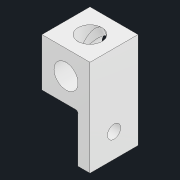
# Autodesk Inventor part: scara-base9
Saved by Autodesk Inventor 2022 (Build 260153000, 153)
## iProperties
Created: 2021-10-21
Part Number: scara-base9
Material: ABS プラスチック
Document SubType Name: Modeling
Designer: Yuta Kage
Density: 1.06 g/cm^3
Appearance: 滑らか - 白
Author: Yuta Kage
Autodesk Inventor part; units mm, degrees
ref_plane "YZ Plane" through (0, 0, 0) normal (1, 0, 0) x (0, 1, 0)
ref_plane "XZ Plane" through (0, 0, 0) normal (0, 1, 0) x (-1, 0, 0)
ref_plane "XY Plane" through (0, 0, 0) normal (0, 0, 1) x (1, 0, 0)
sketch "スケッチ4" plane through (0, 0, 0) normal (0, 0, 1) x (1, 0, 0)
  line L0 (0, 0) -> (0, 40)
  line L1 (0, 40) -> (-20, 40)
  line L2 (-20, 40) -> (-20, 20)
  line L3 (-20, 20) -> (-5, 20)
  line L4 (-5, 20) -> (-5, 0)
  line L5 (-5, 0) -> (0, 0)
  dimension "d32" = 20
  dimension "d33" = 20
  dimension "d34" = 5
  dimension "d58" = 20
  constraints: 12 end point, 5 perpendicular, 1 vertical
  measures "d32" distance of L3.end L4.end
  measures "d33" distance of L1.end L2.end
  measures "d34" distance between parallel lines of L0 L4
  measures "d58" distance of L0.end L1.end
extrude "押し出し2" add sketch "スケッチ4" along normal mid plane 20
sketch "スケッチ5" plane through (0, 0, 10) normal (1, 0, 0) x (0, 0, -1)
  line L0 (20, 0) -> (0, 0) projected
  point P0 (10, 0)
  point P1 (10, 10)
  point P2 (10, 0)
  dimension "d38" = 10
  constraints: 1 midpoint, 1 vertical alignment
  measures "d38" distance of point (10, 0) point (10, 10)
hole "穴3" at (0, 10, 0) direction (-1, 0, 0) diameter 5.5 end through all clearance for "Socket Head Cap Screw" size "M5" standard "Ansi Metric M Profile"
fillet "フィレット3" radius 1 1 edges at (-5, 20, 0)
sketch "スケッチ6" plane through (-20, 40, 10) normal (0, 1, 0) x (1, 0, 0)
  circle A0 centre (10, 10) radius 5
  line L0 (0, 20) -> (0, 0) projected
  line L1 (20, 0) -> (20, 20) projected
  point P0 (20, 10)
  point P1 (20, 10)
  dimension "d47" = 10
  dimension "d48" = 10
  constraints: 1 centre point, 1 horizontal alignment, 1 midpoint
  measures "d47" diameter of A0
  measures "d48" distance from line of L0 A0.centre
extrude "押し出し3" cut sketch "スケッチ6" against normal blind 10
sketch "スケッチ8" plane through (0, 0, 10) normal (0, 0, 1) x (1, 0, 0)
  circle A0 centre (-10, 30) radius 5
  line L0 (0, 40) -> (-20, 40) projected
  line L1 (-20, 40) -> (-20, 20) projected
  point P0 (0, 0)
  dimension "d59" = 10
  dimension "d60" = 10
  dimension "d61" = 10
  constraints: 1 centre point
  measures "d59" diameter of A0
  measures "d60" distance from line of A0.centre L0
  measures "d61" distance from line of L1 A0.centre
extrude "押し出し5" cut sketch "スケッチ8" against normal blind 20
fillet "フィレット6" radius 5 4 edges at (-6.4645, 33.5355, -3.5355) (-13.5355, 33.5355, -3.5355) (-13.5355, 33.5355, 3.5355) (-6.4645, 33.5355, 3.5355)
